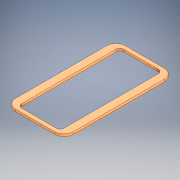
# Autodesk Inventor part: top
Saved by Autodesk Inventor 2020 (Build 240168000, 168)
## iProperties
Created: 2019-11-30
Part Number: top
Material: Bois (cerisier)
Document SubType Name: Modeling
Designer: bapti
Density: 0.63 g/cm^3
Appearance: Cerisier - Faible lustre naturel
Mass: 63.504 g
Surface Area: 436.388 cm^2
Volume: 100.8 cm^3
Author: bapti
Autodesk Inventor part; units mm, degrees
ref_plane "YZ Plane" through (0, 0, 0) normal (1, 0, 0) x (0, 1, 0)
ref_plane "XZ Plane" through (0, 0, 0) normal (0, 1, 0) x (-1, 0, 0)
ref_plane "XY Plane" through (0, 0, 0) normal (0, 0, 1) x (1, 0, 0)
sketch "Esquisse1" plane through (0, 0, 0) normal (0, 1, 0) x (-1, 0, 0)
  line L0 (25, 0) -> (125, 0)
  line L1 (150, -25) -> (150, -260)
  line L2 (125, -285) -> (25, -285)
  line L3 (0, -260) -> (0, -25)
  line L4 (20, 0) -> (20, -10) construction
  line L5 (20, -10) -> (0, -10) construction
  line L6 (150, 0) -> (0, -285) construction
  line L7 (150, -285) -> (0, 0) construction
  line L8 (75, 0) -> (75, -285) construction
  line L9 (150, -142.5) -> (0, -142.5) construction
  line L10 (30, -10) -> (120, -10)
  line L11 (130, -20) -> (130, -265)
  line L12 (120, -275) -> (30, -275)
  line L13 (20, -265) -> (20, -20)
  line L14 (130, -275) -> (150, -275) construction
  line L15 (130, -275) -> (130, -285) construction
  arc A0 (120, -275) -> (130, -265) centre (120, -265) ccw
  arc A1 (20, -265) -> (30, -275) centre (30, -265) ccw
  arc A2 (30, -10) -> (20, -20) centre (30, -20) ccw
  arc A3 (130, -20) -> (120, -10) centre (120, -20) ccw
  arc A4 (25, 0) -> (0, -25) centre (25, -25) ccw
  arc A5 (150, -25) -> (125, 0) centre (125, -25) ccw
  arc A6 (125, -285) -> (150, -260) centre (125, -260) ccw
  arc A7 (0, -260) -> (25, -285) centre (25, -260) ccw
  point P0 (150, -10)
  point P1 (148, 0)
  point P2 (0, -10)
  point P3 (10, 0)
  point P4 (0, -283)
  point P5 (2, -285)
  point P6 (140, -285)
  point P7 (150, -283)
  dimension "d0" = 150
  dimension "d5" = 20
  dimension "d11" = 10
  dimension "d13" = 10
  dimension "d14" = 265
  dimension "d15" = 25
  constraints: 32 end point, 24 point on line, 16 point on circle, 16 tangent, 8 centre point, 6 equal radius, 6 parallel, 5 perpendicular, 4 midpoint, 2 horizontal, 1 vertical
  measures "d0" distance of L7.start L6.end
  measures "d5" distance of L4.end L5.end
  measures "d11" radius of A0
  measures "d13" distance of L4.start L4.end
  measures "d14" distance between parallel lines of L12 L10
  measures "d15" radius of A4
extrude "Extrusion1" add sketch "Esquisse1" along normal blind 6
